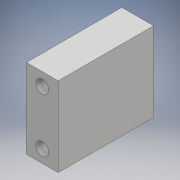
# Autodesk Inventor part: mocowanie uchwytu02
Saved by Autodesk Inventor 2017 (Build 210142000, 142)
## iProperties
Created: 2021-05-23
Part Number: mocowanie uchwytu02
Material: Generic
Document SubType Name: Modeling
Designer: majch
Density: 1 g/cm^3
Appearance: Default
Author: majch
Autodesk Inventor part; units mm, degrees
ref_plane "YZ Plane" through (0, 0, 0) normal (1, 0, 0) x (0, 1, 0)
ref_plane "XZ Plane" through (0, 0, 0) normal (0, 1, 0) x (-1, 0, 0)
ref_plane "XY Plane" through (0, 0, 0) normal (0, 0, 1) x (1, 0, 0)
sketch "Sketch1" plane through (0, 0, 0) normal (0, 1, 0) x (-1, 0, 0)
  line L0 (4, 4) -> (-6, 4)
  line L1 (-6, 4) -> (-6, -21)
  line L2 (-6, -21) -> (4, -21)
  line L3 (4, -21) -> (4, 4)
  point P0 (0, 0)
  dimension "d0" = 10
  dimension "d1" = 25
  constraints: 8 end point, 2 parallel, 1 horizontal, 1 perpendicular
  measures "d0" distance of L2.end L1.end
  measures "d1" distance of L1.end L0.end
extrude "Extrusion1" add sketch "Sketch1" along normal blind 30
sketch "Sketch2" plane through (0, 30, 0) normal (0, 1, 0) x (1, 0, 0)
  line L0 (1, 28) -> (1, -15) construction
  line L1 (-4, 21) -> (-4, -4) projected
  circle A0 centre (1, 17) radius 2
  circle A1 centre (1, 0) radius 2
  line L2 (-4, -4) -> (6, -4) projected
  point P0 (0, 0)
  dimension "d5" = 5
  dimension "d6" = 4
  dimension "d7" = 4
  dimension "d8" = 17
  dimension "d9" = 4
  dimension "d10" = 25
  constraints: 2 centre point, 2 end point, 2 point on line
  measures "d5" distance between parallel lines of L1 L0
  measures "d6" diameter of A0
  measures "d7" diameter of A1
  measures "d8" distance of A1.centre A0.centre
  measures "d9" distance from line of L2 A1.centre
  measures "d10" distance of L1.start L1.end
hole "Hole1" at (1, 30, 0) at (1, 30, -17) direction (0, -1, 0) diameter 4 end through all
equation "\"d9\" = -0.5 * d8 + 0.5 * d10"
body "Solid1"
